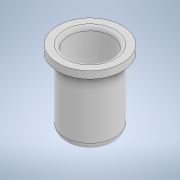
# Autodesk Inventor part: 79. Предохранитель заднего хода
Saved by Autodesk Inventor 2021 (Build 250183000, 183)
## iProperties
Created: 2021-03-15
Part Number: 79. Предохранитель заднего хода
Material: Типовые
Document SubType Name: Modeling
Designer: Данил
Density: 1 g/cm^3
Appearance: По умолчанию
Author: Данил
Autodesk Inventor part; units mm, degrees
ref_plane "YZ Plane" through (0, 0, 0) normal (1, 0, 0) x (0, 1, 0)
ref_plane "XZ Plane" through (0, 0, 0) normal (0, 1, 0) x (-1, 0, 0)
ref_plane "XY Plane" through (0, 0, 0) normal (0, 0, 1) x (1, 0, 0)
sketch "Эскиз1" plane through (0, 0, 0) normal (0, 0, 1) x (1, 0, 0)
  line L0 (0, 11) -> (0, -11)
  arc A0 (0, -11) -> (5.8333, -9.7268) centre (0, 3) ccw
  arc A1 (5.8333, -9.7268) -> (7, -7.9087) centre (5, -7.9087) ccw
  line L1 (7, -7.9087) -> (7, 8)
  line L2 (8, 9) -> (9, 9)
  line L3 (9, 9) -> (9, 11)
  line L4 (9, 11) -> (7, 11)
  arc A2 (8, 9) -> (7, 8) centre (8, 8) ccw
  line L5 (6, 10) -> (6, -3)
  arc A3 (0, -9) -> (6, -3) centre (0, -3) ccw
  arc A4 (7, 11) -> (6, 10) centre (7, 10) ccw
  arc A5 (6, -3) -> (6, -3) centre (8, -3) ccw
  line L6 (0, -9) -> (0, -11)
  point P0 (0, 0)
  point P1 (0, 0)
  point P2 (6, -3)
  dimension "d0" = 22
  dimension "d1" = 14
  dimension "d2" = 2
  dimension "d4" = 14
  dimension "d5" = 1
  dimension "d6" = 18
  dimension "d7" = 1
  dimension "d8" = 2
  dimension "d9" = 2
  dimension "d10" = 2
  dimension "d11" = 1
  constraints: 14 end point, 13 point on circle, 9 tangent, 6 centre point, 4 point on line, 2 perpendicular, 2 vertical, 1 coincident, 1 collinear, 1 horizontal, 1 horizontal alignment, 1 midpoint, 1 parallel
  measures "d0" distance of L0.start L0.end
  measures "d1" radius of A0
  measures "d2" radius of A1
  measures "d4" diameter of L1 L0
  measures "d5" radius of A2
  measures "d6" diameter of L3 L0
  measures "d7" radius of A4
  measures "d8" radius of A5
  measures "d9" distance of L0.end L6.start
  measures "d10" distance of L2.end L3.end
  measures "d11" distance between parallel lines of L5 L1
revolve "Вращение1" add sketch "Эскиз1" angle 360 about axis through (0, 11, 0) along (0, -1, 0) picked at (6.6667, -3) contours A3 A5 L1 A1 A0 L0 | L5 A4 L4 L3 L2 A2 L1 A5 | A5 L1
